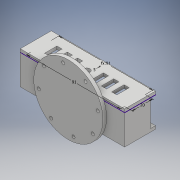
# Autodesk Inventor part: realsense_circle
Saved by Autodesk Inventor 2018 (Build 220112000, 112)
## iProperties
Created: 2018-03-14
Part Number: realsense_circle
Material: Generic
Document SubType Name: Modeling
Designer: Bardo91
Density: 1 g/cm^3
Appearance: Default
Author: Bardo91
Autodesk Inventor part; units mm, degrees
ref_plane "YZ Plane" through (0, 0, 0) normal (1, 0, 0) x (0, 1, 0)
ref_plane "XZ Plane" through (0, 0, 0) normal (0, 1, 0) x (-1, 0, 0)
ref_plane "XY Plane" through (0, 0, 0) normal (0, 0, 1) x (1, 0, 0)
sketch "Sketch1" plane through (0, 0, 0) normal (0, 0, 1) x (1, 0, 0)
  line L0 (0, 0) -> (91, 0)
  line L1 (91, 0) -> (91, 20)
  line L2 (91, 20) -> (0, 20)
  line L3 (0, 20) -> (0, 0)
  line L4 (-5, 25) -> (96, 25)
  line L5 (96, 25) -> (96, -5)
  line L6 (96, -5) -> (-5, -5)
  line L7 (-5, -5) -> (-5, 25)
  line L8 (0, 20) -> (-5, 20)
  line L9 (91, 20) -> (96, 20)
  dimension "d0" = 91
  dimension "d1" = 20
  dimension "d2" = 91
  dimension "d3" = 5
  constraints: 20 end point, 5 perpendicular, 3 point on line, 1 horizontal, 3 other
  measures "d0" distance of L0.start L0.end
  measures "d1" distance of L0.end L1.end
  measures "d2" distance of L1.end L2.end
  measures "d3" distance between parallel lines of L2 L4
extrude "Extrusion1" add sketch "Sketch1" along normal blind 3
extrude "Extrusion2" add sketch "Sketch1" against normal blind 26 contours L0 L1 L9 L5 L6 L7 L8 L3
sketch "Sketch2" plane through (0, 0, -26) normal (0, 0, -1) x (-1, 0, 0)
  line L0 (5, -5) -> (-96, -5) projected
  line L1 (-96, 25) -> (5, 25) projected
  line L2 (-96, -5) -> (5, -5)
  line L3 (5, -5) -> (5, 25)
  line L4 (5, 25) -> (-96, 25)
  line L5 (-96, 25) -> (-96, -5)
  point P0 (0, 0)
  constraints: 8 end point, 2 parallel, 1 horizontal, 1 perpendicular
extrude "Extrusion3" add sketch "Sketch2" along normal blind 3
sketch "Sketch3" plane through (0, 0, 3) normal (0, 0, 1) x (1, 0, 0)
  line L0 (91, 0) -> (0, 0) projected
  line L1 (45.5, 0) -> (45.5, 9)
  circle A0 centre (45.5, 9) radius 3
  dimension "d10" = 9
  dimension "d11" = 6
  constraints: 2 end point, 1 centre point, 1 coincident, 1 midpoint, 1 vertical
  measures "d10" distance of L1.start L1.end
  measures "d11" diameter of A0
extrude "Extrusion4" cut sketch "Sketch3" against normal blind 3
sketch "Sketch6" plane through (-5, -5, 3) normal (0, -1, 0) x (1, 0, 0)
  line L0 (0, -32) -> (101, -32) projected
  line L1 (50.5, -32) -> (50.5, -52)
  line L2 (50.5, -52) -> (56.5, -52)
  line L3 (56.5, -52) -> (56.5, -53.5)
  line L4 (56.5, -53.5) -> (54, -53.5)
  line L5 (54, -53.5) -> (54, -50.5)
  line L6 (54, -50.5) -> (59, -50.5)
  line L7 (59, -50.5) -> (59, -53.5)
  line L8 (59, -53.5) -> (56.5, -53.5)
  line L9 (50.5, -52) -> (44.5, -52)
  line L10 (44.5, -52) -> (44.5, -53.5)
  line L11 (44.5, -53.5) -> (47, -53.5)
  line L12 (47, -53.5) -> (47, -50.5)
  line L13 (47, -50.5) -> (42, -50.5)
  line L14 (42, -50.5) -> (42, -53.5)
  line L15 (42, -53.5) -> (44.5, -53.5)
  point P0 (5, -3)
  dimension "d23" = 20
  dimension "d25" = 6
  dimension "d26" = 1.5
  dimension "d27" = 2.5
  dimension "d28" = 3
  dimension "d29" = 5
  constraints: 30 end point, 6 symmetric about line, 4 perpendicular, 3 vertical, 1 horizontal, 1 midpoint
  measures "d23" distance of L1.start L1.end
  measures "d25" distance of L1.end L2.end
  measures "d26" distance of L2.end L3.end
  measures "d27" distance of L3.end L4.end
  measures "d28" distance of L4.end L5.end
  measures "d29" distance of L5.end L6.end
extrude "Extrusion7" cut sketch "Sketch6" against normal through all
sketch "Sketch7" plane through (0, 0, -26) normal (0, 0, 1) x (1, 0, 0)
  circle A0 centre (39.5, 5) radius 1.5 projected
  circle A1 centre (39.5, 5) radius 3.5
  circle A2 centre (51.5, 5) radius 1.5 projected
  circle A3 centre (51.5, 5) radius 3.5
  dimension "d32" = 7
  dimension "d33" = 7
  constraints: 2 centre point, 2 coincident
  measures "d32" diameter of A1
  measures "d33" diameter of A3
extrude "Extrusion8" cut sketch "Sketch7" against normal blind 10
sketch "Sketch8" plane through (-5, -5, 3) normal (-1, 0, 0) x (0, 0, 1)
  line L0 (-3, 5) -> (-3, 25) projected
  line L1 (-3, 5) -> (-29, 5)
  line L2 (-29, 5) -> (-29, 13)
  line L3 (-29, 13) -> (-3, 13)
  line L4 (-3, 13) -> (-3, 5)
  dimension "d37" = 26
  dimension "d38" = 8
  constraints: 8 end point, 2 parallel, 1 horizontal, 1 perpendicular
  measures "d37" distance of L2.end L3.end
  measures "d38" distance of L1.end L2.end
extrude "Extrusion9" cut sketch "Sketch8" against normal up to surface (5 mm away)
fillet "Fillet2" radius 3 4 edges at (-2.5, 8, 0) (43, 0, 0) (-2.5, 8, -26) (43, 0, -26)
sketch "Sketch9" plane through (0, 0, 3) normal (0, 0, 1) x (1, 0, 0)
  circle A0 centre (45.5, 9) radius 3 projected
  line L0 (45.5, 9) -> (35.5, 9)
  line L1 (35.5, 9) -> (35.5, 15)
  line L2 (35.5, 15) -> (30.5, 15)
  line L3 (30.5, 15) -> (30.5, 3)
  line L4 (35.5, 9) -> (35.5, 3)
  line L5 (35.5, 3) -> (30.5, 3)
  line L6 (30.5, 9) -> (25.5, 9)
  line L7 (25.5, 9) -> (25.5, 15)
  line L8 (25.5, 15) -> (20.5, 15)
  line L9 (20.5, 15) -> (20.5, 3)
  line L10 (20.5, 3) -> (25.5, 3)
  line L11 (25.5, 3) -> (25.5, 9)
  line L12 (20.5, 9) -> (15.5, 9)
  line L13 (15.5, 9) -> (15.5, 15)
  line L14 (15.5, 15) -> (10.5, 15)
  line L15 (10.5, 15) -> (10.5, 3)
  line L16 (10.5, 3) -> (15.5, 3)
  line L17 (15.5, 3) -> (15.5, 9)
  line L18 (45.5, 9) -> (45.5, 56.359)
  line L19 (45.5, 9) -> (55.5, 9)
  line L20 (55.5, 9) -> (55.5, 15)
  line L21 (55.5, 15) -> (60.5, 15)
  line L22 (60.5, 15) -> (60.5, 3)
  line L23 (55.5, 9) -> (55.5, 3)
  line L24 (55.5, 3) -> (60.5, 3)
  line L25 (60.5, 9) -> (65.5, 9)
  line L26 (65.5, 9) -> (65.5, 15)
  line L27 (65.5, 15) -> (70.5, 15)
  line L28 (70.5, 15) -> (70.5, 3)
  line L29 (70.5, 3) -> (65.5, 3)
  line L30 (65.5, 3) -> (65.5, 9)
  line L31 (70.5, 9) -> (75.5, 9)
  line L32 (75.5, 9) -> (75.5, 15)
  line L33 (75.5, 15) -> (80.5, 15)
  line L34 (80.5, 15) -> (80.5, 3)
  line L35 (80.5, 3) -> (75.5, 3)
  line L36 (75.5, 3) -> (75.5, 9)
  point P0 (0, 0)
  point P1 (91, 0)
  dimension "d42" = 10
  dimension "d43" = 6
  dimension "d44" = 5
  dimension "d45" = 12
  dimension "d46" = 6
  dimension "d47" = 5
  dimension "d48" = 6
  dimension "d49" = 5
  dimension "d50" = 12
  dimension "d51" = 5
  dimension "d52" = 5
  dimension "d53" = 6
  dimension "d54" = 5
  dimension "d55" = 12
  dimension "d56" = 5
  constraints: 74 end point, 18 symmetric about line, 14 point on line, 5 perpendicular, 4 vertical, 2 horizontal, 2 midpoint
  measures "d42" distance of L0.start L0.end
  measures "d43" distance of L0.end L1.end
  measures "d44" distance of L1.end L2.end
  measures "d45" distance of L2.end L3.end
  measures "d46" distance of L0.end L4.end
  measures "d47" distance of L6.start L6.end
  measures "d48" distance of L6.end L7.end
  measures "d49" distance of L7.end L8.end
  measures "d50" distance of L8.end L9.end
  measures "d51" distance of L9.end L10.end
  measures "d52" distance of L12.start L12.end
  measures "d53" distance of L12.end L13.end
  measures "d54" distance of L13.end L14.end
  measures "d55" distance of L14.end L15.end
  measures "d56" distance of L15.end L16.end
extrude "Extrusion10" cut sketch "Sketch9" against normal through all contours L17 L16 L15 L14 L13 | L11 L10 L9 L8 L7 | L4 L5 L3 L2 L1 | L32 L33 L34 L35 L36 | L26 L27 L28 L29 L30 | L20 L21 L22 L24 L23
sketch "Sketch12" plane through (-5, -5, 3) normal (0, -1, 0) x (1, 0, 0)
  circle A0 centre (50.05, -16) radius 33.5
  line L0 (0, 0) -> (0, -32) projected
  line L1 (0, 0) -> (101, 0) projected
  point P0 (5, -3)
  dimension "d67" = 67
  dimension "d68" = 50.05
  dimension "d69" = 16
  constraints: 1 centre point
  measures "d67" diameter of A0
  measures "d68" distance from line of L0 A0.centre
  measures "d69" distance from line of L1 A0.centre
extrude "Extrusion12" add sketch "Sketch12" along normal blind 3.5
sketch "Sketch14" plane through (45.05, -8.5, -13) normal (0, -1, 0) x (1, 0, 0)
  circle A0 centre (5.0357, -28.559) radius 1.5
  circle A1 centre (23.7551, -16.6335) radius 1.5
  circle A2 centre (28.559, 5.0357) radius 1.5
  circle A3 centre (16.6335, 23.7551) radius 1.5
  circle A4 centre (-5.0357, 28.559) radius 1.5
  circle A5 centre (-23.7551, 16.6335) radius 1.5
  circle A6 centre (-28.559, -5.0357) radius 1.5
  circle A7 centre (-16.6335, -23.7551) radius 1.5
  point P0 (-45.05, 13)
  point P1 (0, 0)
  dimension "d82" = 3
  dimension "d86" = 360
  constraints: 8 centre point, 17 other
  measures "d82" diameter of A0
extrude "Extrusion14" cut sketch "Sketch14" against normal blind 3.5
equation "\"d2\" = d0"
body "Solid1"
